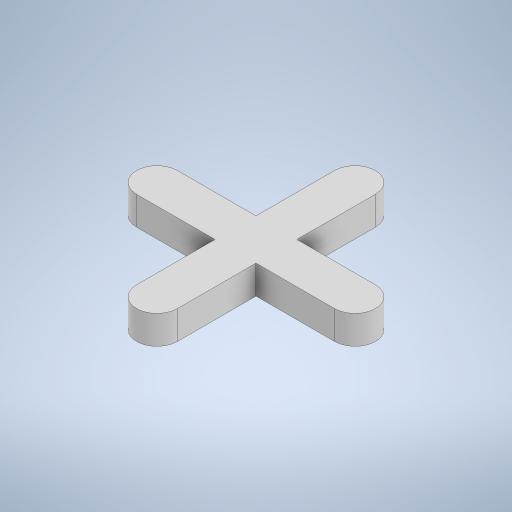
# Autodesk Inventor part: Part7 x 2
Saved by Autodesk Inventor 2023.1 (Build 271208000, 208)
## iProperties
Created: 2022-11-03
Part Number: Part7 x 2
Material: Generic
Document SubType Name: Modeling
Designer: jshin23
Density: 1 g/cm^3
Appearance: Default
Author: jshin23
Autodesk Inventor part; units mm, degrees
ref_plane "YZ Plane" through (0, 0, 0) normal (1, 0, 0) x (0, 1, 0)
ref_plane "XZ Plane" through (0, 0, 0) normal (0, 1, 0) x (-1, 0, 0)
ref_plane "XY Plane" through (0, 0, 0) normal (0, 0, 1) x (1, 0, 0)
sketch "Sketch1" plane through (0, 0, 0) normal (0, 1, 0) x (-1, 0, 0)
  line L0 (0, 0) -> (11.684, 0)
  line L1 (11.684, 0) -> (11.684, -6.096)
  line L2 (11.684, -6.096) -> (0, -6.096)
  line L3 (0, -6.096) -> (0, -17.78)
  line L4 (0, -17.78) -> (-6.096, -17.78)
  line L5 (-6.096, -17.78) -> (-6.096, -6.096)
  line L6 (-6.096, -6.096) -> (-17.78, -6.096)
  line L7 (-17.78, -6.096) -> (-17.78, 0)
  line L8 (-17.78, 0) -> (-6.096, 0)
  line L9 (-6.096, 0) -> (-6.096, 11.684)
  line L10 (-6.096, 11.684) -> (0, 11.684)
  line L11 (0, 11.684) -> (0, 0)
  arc A0 (11.684, -6.096) -> (11.684, 0) centre (11.684, -3.048) ccw
  arc A1 (-6.096, -17.78) -> (0, -17.78) centre (-3.048, -17.78) ccw
  arc A2 (-17.78, 0) -> (-17.78, -6.096) centre (-17.78, -3.048) ccw
  arc A3 (0, 11.684) -> (-6.096, 11.684) centre (-3.048, 11.684) ccw
  dimension "d0" = 11.684
  dimension "d1" = 6.096
  dimension "d2" = 11.684
  dimension "d3" = 6.096
  dimension "d4" = 11.684
  dimension "d5" = 11.684
  constraints: 24 end point, 8 perpendicular, 8 point on circle, 8 tangent, 7 point on line, 4 centre point, 1 horizontal
  measures "d0" distance of L0.start L0.end
  measures "d1" distance of L0.end L1.end
  measures "d2" distance of L2.end L3.end
  measures "d3" distance of L3.end L4.end
  measures "d4" distance of L5.end L6.end
  measures "d5" distance of L8.end L9.end
extrude "Extrusion1" add sketch "Sketch1" along normal blind 4.2418
body "Solid1"
